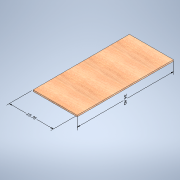
# Autodesk Inventor part: 2020 Wood BaseV04
Saved by Autodesk Inventor 2020.2 (Build 242310000, 310)
## iProperties
Created: 2020-01-12
Part Number: 2020 Wood BaseV04
Material: Wood (Birch)
Document SubType Name: Modeling
Designer: robst
Density: 0.55 g/cm^3
Appearance: Birch - Natural Polished
Author: robst
Autodesk Inventor part; units mm, degrees
ref_plane "YZ Plane" through (0, 0, 0) normal (1, 0, 0) x (0, 1, 0)
ref_plane "XZ Plane" through (0, 0, 0) normal (0, 1, 0) x (-1, 0, 0)
ref_plane "XY Plane" through (0, 0, 0) normal (0, 0, 1) x (1, 0, 0)
sketch "Sketch1" plane through (0, 0, 0) normal (0, 1, 0) x (-1, 0, 0)
  line L0 (200.025, 436.88) -> (-200.025, 436.88)
  line L1 (-200.025, 436.88) -> (-200.025, -436.88)
  line L2 (-200.025, -436.88) -> (200.025, -436.88)
  line L3 (200.025, -436.88) -> (200.025, 436.88)
  line L4 (200.025, 436.88) -> (-200.025, -436.88) construction
  line L5 (-200.025, 436.88) -> (200.025, -436.88) construction
  point P0 (0, 0)
  dimension "d0" = 400.05
  dimension "d1" = 873.76
  constraints: 12 end point, 2 midpoint, 2 parallel, 1 horizontal, 1 perpendicular
  measures "d0" distance of L0.start L0.end
  measures "d1" distance of L1.end L0.end
extrude "Extrusion1" add sketch "Sketch1" along normal blind 12.7
body "Solid1"
